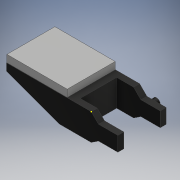
# Autodesk Inventor part: EE Claw
Saved by Autodesk Inventor 2017 (Build 210142000, 142)
## iProperties
Created: 2018-10-18
Part Number: EE Claw
Material: Generic
Document SubType Name: Modeling
Designer: Cameron
Density: 1 g/cm^3
Appearance: Glossy - Black
Author: Cameron
Autodesk Inventor part; units mm, degrees
ref_plane "YZ Plane" through (0, 0, 0) normal (1, 0, 0) x (0, 1, 0)
ref_plane "XZ Plane" through (0, 0, 0) normal (0, 1, 0) x (-1, 0, 0)
ref_plane "XY Plane" through (0, 0, 0) normal (0, 0, 1) x (1, 0, 0)
sketch "Sketch1" plane through (0, 0, 0) normal (0, 1, 0) x (-1, 0, 0)
  point P0 (0, 0)
sketch "Sketch2" plane through (0, 0, 0) normal (0, 1, 0) x (-1, 0, 0)
  line L0 (0, 0) -> (35, 0)
  line L1 (35, 0) -> (35, -3)
  line L2 (13, -11) -> (35, -3)
  line L3 (13, -11) -> (0, -11)
  line L4 (-3, -9) -> (0, -11)
  line L5 (-3, -9) -> (-11, -9)
  line L6 (-11, -9) -> (-11, -3)
  line L7 (-11, -3) -> (-3, -3)
  line L8 (-3, -3) -> (0, 0)
  dimension "d0" = 35
  dimension "d1" = 3
  dimension "d8" = 6
  constraints: 18 end point, 3 perpendicular, 2 horizontal
  measures "d0" distance of L0.start L0.end
  measures "d1" distance of L0.end L1.end
  measures "d8" distance of L5.end L6.end
extrude "Extrusion1" add sketch "Sketch2" along normal blind 20
sketch "Sketch3" plane through (0, 20, 0) normal (0, 1, 0) x (1, 0, 0)
  line L0 (11, 9) -> (11, 3) projected
  line L1 (11, 6) -> (4, 6)
  circle A0 centre (4, 6) radius 1.5
  dimension "d11" = 7
  dimension "d12" = 3
  constraints: 2 end point, 1 centre point, 1 coincident, 1 horizontal, 1 midpoint
  measures "d11" distance of L1.start L1.end
  measures "d12" diameter of A0
extrude "Extrusion2" add sketch "Sketch3" along normal blind 3
sketch "Sketch4" plane through (-35, 0, 0) normal (0, 0, 1) x (1, 0, 0)
  line L0 (46, 0) -> (46, 20) projected
  line L1 (46, 10) -> (28, 10)
  line L2 (28, 10) -> (28, 17.5)
  line L3 (28, 17.5) -> (28, 2.5)
  line L4 (28, 2.5) -> (46, 2.5)
  line L5 (28, 17.5) -> (46, 17.5)
  line L6 (46, 2.5) -> (46, 17.5)
  dimension "d15" = 18
  dimension "d16" = 7.5
  dimension "d17" = 15
  constraints: 12 end point, 3 perpendicular, 3 point on line, 1 horizontal, 1 midpoint, 1 parallel
  measures "d15" distance of L1.start L1.end
  measures "d16" distance of L1.end L2.end
  measures "d17" distance of L2.end L3.end
extrude "Extrusion3" cut sketch "Sketch4" against normal through all
sketch "Sketch5" plane through (-35, 0, 0) normal (0, 0, 1) x (1, 0, 0)
  line L0 (28, 17.5) -> (35, 17.5) projected
  line L1 (35, 17.5) -> (35, 20) projected
  line L2 (0, 20) -> (35, 20) projected
  line L3 (35, 0) -> (35, 2.5) projected
  line L4 (35, 2.5) -> (28, 2.5) projected
  line L5 (28, 2.5) -> (28, 17.5) projected
  line L6 (0, 0) -> (25, 0)
  line L7 (25, 0.1) -> (25, 19.9)
  line L8 (25, 20) -> (0, 20)
  line L9 (0, 20) -> (0, 0)
  line L10 (34.9, 19.9) -> (34.9, 17.6)
  line L11 (34.9, 17.6) -> (27.9, 17.6)
  line L12 (27.9, 17.6) -> (27.9, 2.4)
  line L13 (27.9, 2.4) -> (34.9, 2.4)
  line L14 (34.9, 2.4) -> (34.9, 0.1)
  line L15 (25, 0.1) -> (0.1, 0.1)
  line L16 (0.1, 0.1) -> (0.1, 19.9)
  line L17 (0.1, 19.9) -> (25, 19.9)
  dimension "d20" = 25
  dimension "d21" = 0.1
  constraints: 24 end point, 2 parallel, 1 horizontal, 1 perpendicular, 1 point on line, 4 other
  measures "d20" distance of L8.end L8.start
  measures "d21" distance between parallel lines of L2 L17
extrude "Extrusion4" add sketch "Sketch5" along normal blind 3
body "Solid1"
